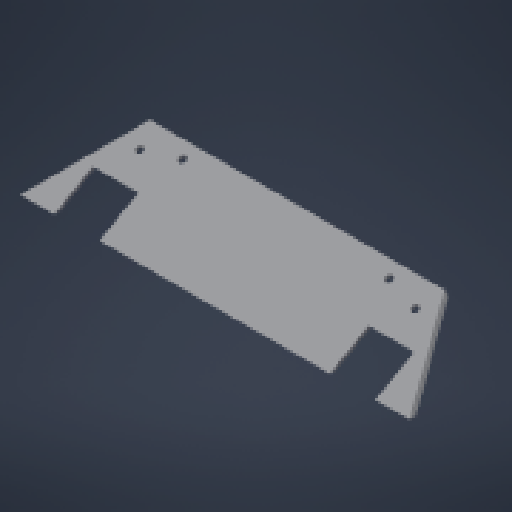
# Autodesk Inventor part: Przod2mm
Saved by Autodesk Inventor 2023 (Build 270158000, 158)
## iProperties
Created: 2022-01-22
Part Number: Przod2mm
Material: Ogólny
Document SubType Name: Modeling
Designer: Michał
Density: 1 g/cm^3
Appearance: Domyślna
Author: Michał
Autodesk Inventor part; units mm, degrees
ref_plane "YZ Plane" through (0, 0, 0) normal (1, 0, 0) x (0, 1, 0)
ref_plane "XZ Plane" through (0, 0, 0) normal (0, 1, 0) x (-1, 0, 0)
ref_plane "XY Plane" through (0, 0, 0) normal (0, 0, 1) x (1, 0, 0)
sketch "Szkic1" plane through (0, 0, 0) normal (1, 0, 0) x (0, 1, 0)
  line L0 (0.433, -0.75) -> (22.433, -38.8551)
  line L1 (22.433, -38.8551) -> (21.134, -39.6051)
  line L2 (21.134, -39.6051) -> (0.433, -3.75)
  line L3 (0.433, -3.75) -> (0.433, -0.75)
  line L4 (21.134, -39.6051) -> (21.134, -39.6051)
  dimension "d0" = 1.5
  dimension "d1" = 22
  dimension "d2" = 30
  constraints: 10 end point, 1 coincident, 1 collinear, 1 parallel, 1 perpendicular, 1 point on line, 1 vertical, 1 other
  measures "d0" distance between parallel lines of L2 L0
  measures "d1" distance from line of L3 L0.end
  measures "d2" angle of L3 L2
extrude "Wyciągnięcie proste1" add sketch "Szkic1" along normal blind 180.175
sketch "Szkic2" plane through (180.175, 22.433, 0) normal (0, 0, -1) x (-1, 0, 0)
  line L0 (143.375, -22) -> (164.375, -22)
  line L1 (164.375, -22) -> (164.375, -11.7)
  line L2 (164.375, -11.7) -> (143.375, -11.7)
  line L3 (143.375, -11.7) -> (143.375, -22)
  line L4 (180.175, -22) -> (0, -22) construction
  line L5 (180.175, -22) -> (180.175, 0) construction
  line L6 (180.175, -22) -> (180.175, 0)
  line L7 (180.175, 0) -> (0, 0) construction
  line L8 (158.175, 0) -> (180.175, -22)
  line L9 (90.0875, -22) -> (90.0875, 0) construction
  line L10 (180.175, 0) -> (158.175, 0)
  line L11 (36.8, -22) -> (15.8, -22)
  line L12 (15.8, -22) -> (15.8, -11.7)
  line L13 (15.8, -11.7) -> (36.8, -11.7)
  line L14 (36.8, -11.7) -> (36.8, -22)
  line L15 (0, -22) -> (0, 0) construction
  line L16 (0, -22) -> (0, 0)
  line L17 (22, 0) -> (0, -22)
  line L18 (0, 0) -> (22, 0)
  dimension "d9" = 21
  dimension "d10" = 10.3
  dimension "d33" = 15.8
  dimension "d34" = 45
  constraints: 32 end point, 5 symmetric about line, 2 collinear, 2 midpoint, 2 parallel, 1 horizontal, 1 perpendicular, 1 point on line, 1 vertical
  measures "d9" distance of L0.end L0.start
  measures "d10" distance of L2.end L0.start
  measures "d33" distance between parallel lines of L5 L1
  measures "d34" angle of L5 L8
extrude "Wyciągnięcie proste2" cut sketch "Szkic2" along normal through all
sketch "Szkic3" plane through (22, 22, -38.1051) normal (0, 0.866, 0.5) x (1, 0, 0)
  line L0 (-2, -0.5359) -> (138.175, -0.5359) construction
  line L1 (-2, -0.5359) -> (4.3275, -0.5359) construction
  line L2 (4.3275, -0.5359) -> (4.3275, -10.5359) construction
  line L3 (-2, -0.5359) -> (20.3275, -0.5359) construction
  line L4 (20.3275, -0.5359) -> (20.3275, -6.1359) construction
  line L5 (0, 0.4641) -> (136.175, 0.4641) construction
  line L6 (68.0875, 0.4641) -> (68.0854, -43.134) construction
  line L7 (-22, -43.134) -> (158.175, -43.134) construction
  circle A0 centre (20.3275, -6.1359) radius 1.6
  circle A1 centre (4.3275, -10.5359) radius 1.6
  circle A2 centre (131.8464, -10.542) radius 1.6
  circle A3 centre (115.8469, -6.1405) radius 1.6
  point P0 (-22, -44)
  point P1 (14.8, -43.134)
  point P2 (121.375, -44)
  dimension "d12" = 6.3275
  dimension "d13" = 10
  dimension "d14" = 22.3275
  dimension "d15" = 5.6
  dimension "d16" = 3.2
  dimension "d17" = 3.2
  constraints: 10 end point, 4 centre point, 2 coincident, 2 point on line, 2 vertical, 1 midpoint, 4 other
  measures "d12" distance of L0.start L1.end
  measures "d13" distance of L1.end L2.end
  measures "d14" distance of L3.end L0.start
  measures "d15" distance of L3.end L4.end
  measures "d16" diameter of A0
  measures "d17" diameter of A1
extrude "Wyciągnięcie proste3" cut sketch "Szkic3" against normal through all
